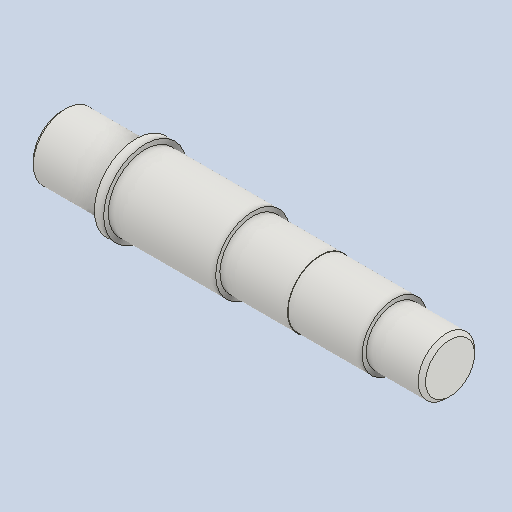
# Autodesk Inventor part: Shaft
Saved by Autodesk Inventor 2025.2 (Build 292293000, 293)
## iProperties
Created: 2024-11-26
Part Number: Shaft
Material: Steel
Document SubType Name: Modeling
Designer: hongquan
Density: 1 g/cm^3
Appearance: Steel
CustomPartVersion: 1
Author: hongquan
Length: 209.500 mm
Autodesk Inventor part; units mm, degrees
ref_plane "Start Plane" through (0, 0, 0) normal (1, 0, 0) x (0, 1, 0)
ref_plane "XZ Plane" through (0, 0, 0) normal (0, 1, 0) x (-1, 0, 0)
ref_plane "XY Plane" through (0, 0, 0) normal (0, 0, 1) x (1, 0, 0)
sketch "Main Sketch" plane through (0, 0, 0) normal (0, 0, 1) x (1, 0, 0)
  line L0 (0, 0) -> (209.5, 0)
  line L1 (0, 0) -> (0, 17.5)
  line L2 (0, 17.5) -> (40, 17.5)
  line L3 (40, 17.5) -> (40, 22.5)
  line L4 (45, 22.5) -> (45, 20)
  line L5 (40, 22.5) -> (45, 22.5)
  line L6 (103, 20) -> (103, 17.75)
  line L7 (45, 20) -> (103, 20)
  line L8 (139.5, 17.75) -> (139.5, 17.5)
  line L9 (103, 17.75) -> (139.5, 17.75)
  line L10 (179.5, 17.5) -> (179.5, 15.25)
  line L11 (139.5, 17.5) -> (179.5, 17.5)
  line L12 (209.5, 15.25) -> (209.5, 0)
  line L13 (179.5, 15.25) -> (209.5, 15.25)
  dimension "d3" = 35
  dimension "d4" = 45
  dimension "d5" = 40
  dimension "d6" = 35.5
  dimension "d7" = 35
  dimension "d8" = 30.5
  constraints: 28 end point, 8 horizontal, 7 vertical
  measures "d3" diameter of L2 L0
  measures "d4" diameter of L5 L0
  measures "d5" diameter of L7 L0
  measures "d6" diameter of L9 L0
  measures "d7" diameter of L11 L0
  measures "d8" diameter of L13 L0
revolve "Revolution1" add sketch "Main Sketch" angle 360 about axis through (0, 0, 0) along (1, 0, 0)
chamfer "Chamfer1" distance 2 angle 45 1 edges at (0, -17.5, 0) measured on face at (26.6667, 17.4433, -1.4082)
chamfer "Chamfer2" distance 2 angle 45 1 edges at (209.5, -15.25, 0) measured on face at (199.5, 15.2005, -1.2271)
equation "\"Length\" = 209.5"
body "Solid1"
